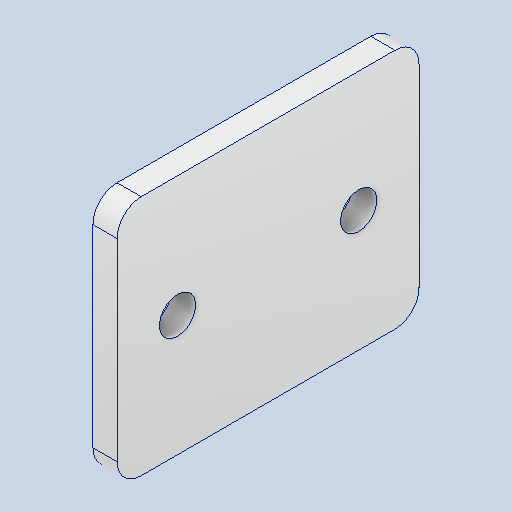
# Autodesk Inventor part: base_weel-v1-Plate-expand-2
Saved by Autodesk Inventor 2025.1 (Build 291241000, 241)
## iProperties
Created: 2024-12-09
Part Number: base_weel-v1-Plate-expand-2
Material: アルミニウム 6061
Document SubType Name: Modeling
Designer: haruy
Density: 2.7 g/cm^3
Appearance: アルミニウム - フラット
Author: haruy
Autodesk Inventor part; units mm, degrees
ref_plane "YZ Plane" through (0, 0, 0) normal (1, 0, 0) x (0, 1, 0)
ref_plane "XZ Plane" through (0, 0, 0) normal (0, 1, 0) x (-1, 0, 0)
ref_plane "XY Plane" through (0, 0, 0) normal (0, 0, 1) x (1, 0, 0)
sketch "スケッチ1" plane through (0, 0, 0) normal (1, 0, 0) x (0, 1, 0)
  line L0 (68.2079, 642.9582) -> (68.2079, -632.5418)
  circle A0 centre (78.2079, 14.9582) radius 1.5
  line L1 (88.2079, -632.5418) -> (68.2079, -632.5418)
  circle A1 centre (78.2079, -0.0418) radius 1.5
  circle A2 centre (78.2079, 14.9582) radius 1.5
  line L2 (68.2079, -5.0418) -> (88.2079, -5.0418)
  line L3 (68.2079, 19.9582) -> (88.2079, 19.9582)
  line L4 (87.2079, 642.9582) -> (87.2079, 7.4582)
  line L5 (68.2079, 19.9582) -> (68.2079, -5.0418)
  line L6 (88.2079, 19.9582) -> (88.2079, -5.0418)
  line L7 (88.2079, 642.9582) -> (88.2079, -632.5418)
  point P0 (0, 0)
  point P1 (-76.7921, 17.4582)
  point P2 (78.2079, -625.0418)
  dimension "d0" = 10
  dimension "d1" = 15
  dimension "d2" = 7.5
  dimension "d3" = 10
  dimension "d4" = 3
  dimension "d5" = 3
  dimension "d6" = 5
  dimension "d7" = 5
  constraints: 16 end point, 3 centre point, 2 coincident, 2 collinear, 2 point on line, 1 horizontal, 1 perpendicular
  measures "d0" distance from line of L0 point (78.208, -0.042)
  measures "d1" distance of A0.centre point (78.208, -0.042)
  measures "d2" distance from line of point (78.208, -625.042) L1
  measures "d3" distance from line of L0 point (78.208, -625.042)
  measures "d4" diameter of A1
  measures "d5" diameter of A2
  measures "d6" distance from line of L2 A1.centre
  measures "d7" distance from line of A0.centre L3
extrude "押し出し1" add sketch "スケッチ1" against normal blind 2 contours L3 L6 L2 L0
fillet "フィレット1" radius 2 4 edges at (-1, 88.2079, 19.9582) (-1, 68.2079, 19.9582) (-1, 88.2079, -5.0418) (-1, 68.2079, -5.0418)
